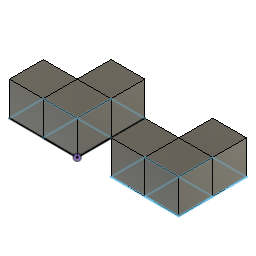
BooleanOverlapDouble (Autodesk Fusion 360 design; units mm, degrees)
Autodesk Fusion 360 part; units mm, degrees
sketch "Sketch1" plane through (0, 0, 0) normal (0, 0, 1) x (1, 0, 0)
  line L0 (0, 0) -> (-20, 0)
  line L1 (-20, 0) -> (-20, 10)
  line L2 (-20, 10) -> (0, 10)
  line L3 (0, 10) -> (0, 0)
  line L4 (0, 0) -> (-10, 0)
  line L5 (-10, 0) -> (-10, 20)
  line L6 (-10, 20) -> (0, 20)
  line L7 (0, 20) -> (0, 0)
  line L8 (10, 10) -> (30, 10)
  line L9 (30, 10) -> (30, 0)
  line L10 (30, 0) -> (10, 0)
  line L11 (10, 0) -> (10, 10)
  line L12 (30, 0) -> (20, 0)
  line L13 (20, 0) -> (20, 20)
  line L14 (20, 20) -> (30, 20)
  line L15 (30, 20) -> (30, 0)
  constraint horizontal L0
  constraint vertical L1
  constraint horizontal L2
  constraint vertical L3
  constraint coincident L0.start L3.end
  constraint horizontal L4
  constraint vertical L5
  constraint horizontal L6
  constraint vertical L7
  constraint horizontal L8
  constraint vertical L9
  constraint horizontal L10
  constraint vertical L11
  constraint horizontal L12
  constraint vertical L13
  constraint horizontal L14
  constraint vertical L15
extrude "Extrude1" add sketch "Sketch1" along normal blind 10 contours L0 L2 L3 L4 L5 L7 | L0 L1 L2 L5 | L8 L10 L11 L13 | L8 L9 L10 L12 L13 L15 makes body 1 at (-13.3333, 3.3333, 0) makes body 2 at (16.6667, 3.3333, 0)
extrude "Extrude2" add sketch "Sketch1" along normal blind 10 separate body contours L0 L2 L3 L4 L5 L7 | L2 L5 L6 L7 | L8 L13 L14 L15 | L8 L9 L10 L12 L13 L15 makes body 3 at (-6.6667, 6.6667, 0) makes body 4 at (23.3333, 6.6667, 0)
